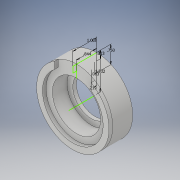
# Autodesk Inventor part: Lower die 2 oweder ring
Saved by Autodesk Inventor 2017.1 (Build 211199000, 199)
## iProperties
Created: 2017-04-14
Part Number: Lower die 2 oweder ring
Material: Generic
Document SubType Name: Modeling
Designer: 196918
Density: 1 g/cm^3
Appearance: Default
Author: 196918
Autodesk Inventor part; units mm, degrees
ref_plane "YZ Plane" through (0, 0, 0) normal (1, 0, 0) x (0, 1, 0)
ref_plane "XZ Plane" through (0, 0, 0) normal (0, 1, 0) x (-1, 0, 0)
ref_plane "XY Plane" through (0, 0, 0) normal (0, 0, 1) x (1, 0, 0)
sketch "Sketch1" plane through (0, 0, 0) normal (1, 0, 0) x (0, 1, 0)
  line L0 (7.148, 22.3374) -> (0.4434, 22.3374)
  line L1 (0.4434, 22.3374) -> (0.4434, 6.4624)
  line L2 (0.4434, 6.4624) -> (-5.5806, 6.4624)
  line L3 (-5.5806, 6.4624) -> (-5.5806, 2.4873)
  line L4 (-5.5806, 2.4873) -> (5.5319, 2.4873)
  line L5 (5.5319, 2.4873) -> (5.5319, 0.8998)
  line L6 (5.5319, 0.8998) -> (13.4694, 0.8998)
  line L7 (7.148, 22.3374) -> (7.1466, 26.2987)
  line L8 (7.1466, 26.2987) -> (13.468, 26.2998)
  line L9 (13.468, 26.2998) -> (13.4694, 22.3374)
  line L10 (13.4694, 22.3374) -> (13.4694, 0.8998)
  line L11 (13.4694, 0.8998) -> (-25.4371, 0.8998) construction
  line L12 (-25.4371, 0.8998) -> (-25.4371, 30.7501)
  line L13 (7.148, 22.3374) -> (13.4694, 22.3374)
  point P0 (0, 0)
  dimension "d7" = 19.05
  dimension "d8" = 7.9375
  dimension "d9" = 5.5626
  dimension "d10" = 1.5875
  dimension "d11" = 25.4
  dimension "d12" = 21.4376
  dimension "d13" = 38.9064
  constraints: 28 end point, 4 horizontal, 4 perpendicular, 2 parallel, 2 vertical
  measures "d7" horizontal distance of L6.end L3.end
  measures "d8" distance of L6.end L5.end
  measures "d9" vertical distance of L6.end L1.end
  measures "d10" distance of L5.end L4.end
  measures "d11" distance of L6.end L8.end
  measures "d12" vertical distance of L6.end L0.start
  measures "d13" distance of L6.end L11.end
revolve "Revolution1" add sketch "Sketch1" angle 360 about axis through (0, -25.4371, 0.8998) along (0, 0, 1) contours L13 L10 L6 L5 L4 L3 L2 L1 L0
revolve "Revolution2" add sketch "Sketch1" angle 360 about axis through (0, -25.4371, 0.8998) along (0, 0, -1) contours L7 L8 L9 L13
sketch "Sketch3" plane through (0, -25.4371, 22.3374) normal (0, 0, 1) x (1, 0, 0)
  line L0 (0, 49.6302) -> (19.8438, 49.6302)
  line L1 (19.8438, 49.6302) -> (-19.8438, 49.6302)
  line L2 (-19.8438, 49.6302) -> (-19.8438, 12.1467)
  line L3 (-19.8438, 12.1467) -> (19.8438, 12.1467)
  line L4 (19.8438, 12.1467) -> (19.8438, 49.6302)
  point P0 (0, 25.4371)
  dimension "d18" = 19.8438
  dimension "d19" = 39.6875
  constraints: 10 end point, 2 horizontal, 2 parallel, 1 perpendicular
  measures "d18" distance of L0.start L0.end
  measures "d19" distance of L3.end L2.end
extrude "Extrusion1" cut sketch "Sketch3" along normal blind 15.875
body "Solid1"
